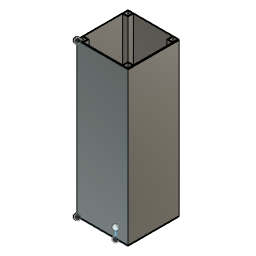
einsat-3u-telescope-v3 (Autodesk Fusion 360 design; units mm, degrees)
Autodesk Fusion 360 part; units mm, degrees
sketch "Sketch1" plane through (0, 0, 0) normal (0, 0, 1) x (1, 0, 0)
  line L0 (-50, 50) -> (50, 50)
  line L1 (50, 50) -> (50, -50)
  line L2 (50, -50) -> (-50, -50)
  line L3 (-50, -50) -> (-50, 50)
  constraint horizontal L0
  constraint vertical L1
  constraint horizontal L2
  constraint vertical L3
extrude "Extrude1" add sketch "Sketch1" along normal blind 1.5 makes body 1
surface "Extrude2" add extruded along (0, 0, 1) between 0 and 297 1 faces at (-16.6667, 16.6667, 1.5) separate body on bodies 1 makes body 2
extrude "Extrude3" add 1 faces at (-16.6667, 50, 100.5) along direction (0, -1, 0) blind 1.5 on bodies 2 bodies 1
extrude "Extrude4" cut 1 faces at (-50, -16.6667, 100.5) along direction (1, 0, 0) blind 1.5 on bodies 2 bodies 1
extrude "Extrude5" add 1 faces at (-50, -16.6667, 100.5) along direction (1, 0, 0) blind 1.5 on bodies 2 bodies 1
extrude "Extrude6" cut 1 faces at (16.6667, -50, 100.5) along direction (0, 1, 0) blind 1.5 on bodies 2 bodies 1
extrude "Extrude7" add 1 faces at (16.6667, -50, 100.5) along direction (0, 1, 0) blind 1.5 on bodies 2 bodies 1
extrude "Extrude8" cut 1 faces at (50, 16.6667, 100.5) along direction (-1, 0, 0) blind 1.5 on bodies 2 bodies 1
extrude "Extrude9" add 1 faces at (50, 16.6667, 100.5) along direction (-1, 0, 0) blind 1.5 on bodies 2 bodies 1
surface "SurfacePatch1" add patch along 4 edges at (0, 50, 298.5) (-50, 0, 298.5) (0, -50, 298.5) (50, 0, 298.5) separate body on bodies 2 makes body 3
delete_face "SurfaceDeleteFace1" leaving the opening 1 faces at (-16.6667, 16.6667, 298.5) on bodies 3
hole "Hole1" at (0, 0, 1.5) direction (0, 0, -1) diameter 76 depth 1.5 tip angle 118 bodies 1
sketch "Sketch2" plane through (0, -50, 0) normal (0, -1, 0) x (1, 0, 0)
  line L0 (50, 298.5) -> (-50, 298.5)
  line L1 (-50, 298.5) -> (-50, 0)
  line L2 (-50, 0) -> (50, 0)
  line L3 (50, 0) -> (50, 298.5)
  line L4 (26, 0) -> (26, 20)
  line L5 (-50, 0) -> (-48.5, 0)
  line L6 (-50, 298.5) -> (-48.5, 298.5)
  constraint coincident L2 L4.start
  constraint perpendicular L2 L4
  constraint coincident L1.end L2.start
  constraint coincident L2 L5.end
  constraint perpendicular L1 L5
  constraint coincident L0 L6.end
  constraint coincident L0.end L1.start
surface "SurfacePatch2" add patch along 4 edges at (-50, 0, 298.5) (0, 50, 298.5) (50, 0, 298.5) (0, -50, 298.5) separate body on bodies 1 makes body 4
extrude "Extrude10" add 1 faces at (16.6667, 16.6667, 298.5) along direction (0, 0, 1) blind 1.5 on bodies 4 bodies 1
sketch "Sketch3" plane through (0, 0, 300) normal (0, 0, 1) x (-1, 0, 0)
  line L0 (50, -50) -> (50, 50)
  line L1 (50, 50) -> (-50, 50)
  line L2 (-50, 50) -> (-50, -50)
  line L3 (-50, -50) -> (50, -50)
  line L4 (50, 50) -> (50, 48.5)
  line L5 (50, 48.5) -> (-50, 48.5)
  line L6 (50, 50) -> (48.5, 50)
  line L7 (-50, 50) -> (-48.5, 50)
  line L8 (-48.5, 50) -> (-48.5, -50)
  line L9 (-50, -50) -> (-50, -48.5)
  line L10 (-50, -48.5) -> (50, -48.5)
  line L11 (48.5, 50) -> (48.5, -50)
  line L12 (48.5, 50) -> (39.5, 50)
  line L13 (39.5, 50) -> (39.5, -50)
  line L14 (39.5, 50) -> (38, 50)
  line L15 (38, 50) -> (38, -50)
  line L16 (50, 48.5) -> (50, 39.5)
  line L17 (50, 39.5) -> (-50, 39.5)
  line L18 (50, 39.5) -> (50, 38)
  line L19 (50, 38) -> (-50, 38)
  line L20 (-48.5, 50) -> (-39.5, 50)
  line L21 (-39.5, 50) -> (-39.5, -50)
  line L22 (-39.5, 50) -> (-38, 50)
  line L23 (-38, 50) -> (-38, -50)
  line L24 (-50, -48.5) -> (-50, -39.5)
  line L25 (-50, -39.5) -> (50, -39.5)
  line L26 (-50, -39.5) -> (-50, -38)
  line L27 (-50, -38) -> (50, -38)
  line L28 (-39.5, -48.5) -> (-48.5, -48.5)
  line L29 (-48.5, -48.5) -> (-48.5, -39.5)
  line L30 (-48.5, -39.5) -> (-39.5, -39.5)
  line L31 (-39.5, -39.5) -> (-39.5, -48.5)
  dimension "d25" = 1.5
  dimension "d26" = 100
  dimension "d27" = 1.5
  dimension "d29" = 1.5
  dimension "d30" = 100
  dimension "d31" = 1.5
  dimension "d32" = 100
  dimension "d33" = 100
  dimension "d34" = 9
  dimension "d35" = 100
  dimension "d36" = 100
  dimension "d37" = 9
  dimension "d38" = 100
  dimension "d39" = 100
  dimension "d40" = 9
  dimension "d41" = 100
  dimension "d42" = 100
  dimension "d43" = 9
  dimension "d44" = 100
  dimension "d45" = 100
  constraint coincident L0.end L1.start
  constraint perpendicular L1 L4
  constraint perpendicular L0 L5
  constraint perpendicular L0 L6
  constraint coincident L1.end L2.start
  constraint perpendicular L2 L7
  constraint perpendicular L5 L8
  constraint coincident L2.end L3.start
  constraint perpendicular L3 L9
  constraint perpendicular L9 L10
  constraint perpendicular L5 L11
  constraint perpendicular L11 L12
  constraint perpendicular L5 L13
  constraint coincident L1 L14.end
  constraint perpendicular L13 L14
  constraint perpendicular L5 L15
  constraint perpendicular L5 L16
  constraint perpendicular L15 L17
  constraint coincident L0 L18.end
  constraint perpendicular L17 L18
  constraint perpendicular L15 L19
  constraint perpendicular L8 L20
  constraint perpendicular L5 L21
  constraint coincident L1 L22.end
  constraint perpendicular L21 L22
  constraint perpendicular L5 L23
  constraint perpendicular L10 L24
  constraint perpendicular L23 L25
  constraint coincident L2 L26.end
  constraint perpendicular L8 L27
  constraint horizontal L28
  constraint vertical L29
  constraint horizontal L30
  constraint vertical L31
  constraint coincident L8 L29.end
  constraint coincident L25 L29.end
  constraint coincident L21 L28.start
  constraint coincident L10 L28.start
  measures "d25" distance of L0.end L4.end
  measures "d26" distance of L4.end L5.end
  measures "d27" distance of L0.end L6.end
  measures "d29" distance of L1.end L7.end
  measures "d30" distance of L7.end L8.end
  measures "d31" distance of L2.end L9.end
  measures "d32" distance of L9.end L10.end
  measures "d33" distance of L6.end L11.end
  measures "d34" distance of L6.end L12.end
  measures "d35" distance of L12.end L13.end
  measures "d36" distance of L14.end L15.end
  measures "d37" distance of L4.end L16.end
  measures "d38" distance of L16.end L17.end
  measures "d39" distance of L18.end L19.end
  measures "d40" distance of L7.end L20.end
  measures "d41" distance of L20.end L21.end
  measures "d42" distance of L22.end L23.end
  measures "d43" distance of L9.end L24.end
  measures "d44" distance of L24.end L25.end
  measures "d45" distance of L26.end L27.end
extrude "Extrude11" cut sketch "Sketch3" against normal blind 1.5 contours L10 L11 L13 L25 | L11 L13 L19 L27 | L10 L15 L23 L25 | L13 L15 L19 L27 | L15 L23 L25 L27 | L5 L11 L13 L17 | L15 L19 L23 L27 | L8 L10 L21 L25 L28 L29 L30 L31 | L15 L17 L19 L23 | L19 L21 L23 L27 | L5 L15 L17 L23 | L8 L19 L21 L27 | L5 L8 L17 L21 bodies 1
delete_face "SurfaceDeleteFace2" leaving the opening 1 faces at (16.6667, 16.6667, 298.5) on bodies 4
extrude "Extrude12" add 4 faces at (42, -38.5, 298.5) (-38.5, -42, 298.5) (42, 38.5, 298.5) (-42, 38.5, 298.5) along direction (0, 0, -1) blind 297 on bodies 1 bodies 1
extrude "Extrude13" cut 4 faces at (-42.5, -42.5, 1.5) (-42.5, 45.5, 1.5) (45.5, 45.5, 1.5) (45.5, -42.5, 1.5) along direction (0, 0, -1) blind 1.5 on bodies 1 bodies 1
